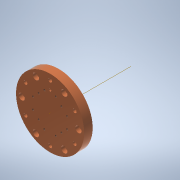
# Autodesk Inventor part: base_becherboden
Saved by Autodesk Inventor 2020 (Build 240168000, 168)
## iProperties
Created: 2018-08-22
Part Number: base_becherboden
Material: ABS Plastic
Document SubType Name: Modeling
Designer: Q
Density: 1.06 g/cm^3
Appearance: Smooth - White
Mass: 1439.4 g
Surface Area: 317.494 cm^2
Volume: 161.006 cm^3
Author: Q
Autodesk Inventor part; units mm, degrees
ref_plane "YZ Plane" through (0, 0, 0) normal (1, 0, 0) x (0, 1, 0)
ref_plane "XZ Plane" through (0, 0, 0) normal (0, 1, 0) x (-1, 0, 0)
ref_plane "XY Plane" through (0, 0, 0) normal (0, 0, 1) x (1, 0, 0)
sketch "Sketch1" plane through (0, 0, 0) normal (0, 0, 1) x (1, 0, 0)
  circle A0 centre (0, 0) radius 60 projected
  point P0 (0, 0)
  point P1 (-51.3571, -31.5041)
  point P2 (-31.5041, -51.3571)
  constraints: 1 other
extrude "Extrusion1" add sketch "Sketch1" along normal blind 15
sketch "Sketch13" plane through (0, 0, 0) normal (0, 0, -1) x (-1, 0, 0)
  point P0 (0, 0)
  point P1 (0, 0)
  constraints: 1 coincident
sketch "Sketch14" plane through (0, 0, 15) normal (0, 0, 1) x (1, 0, 0)
  circle A0 centre (0, 50) radius 2.4585 projected
  point P0 (0, 0)
hole "Hole10" at (0, 50, 15) direction (0, 0, -1) diameter 6.6 depth 17.1 clearance for "Socket Head Cap Screw ISO 4762" size "M6" standard "ISO"
pattern_circular "Circular Pattern6" count 6 over 360 about axis through (0, 0, 0) along (0, 0, 1) of "Hole10"
sketch "Sketch15" plane through (0, 0, 15) normal (0, 0, 1) x (1, 0, 0)
  circle A0 centre (25, 43.3013) radius 2.4585 projected
  point P0 (0, 0)
hole "Hole11" at (25, 43.3013, 15) direction (0, 0, -1) diameter 6.6 end through all counterbore diameter 11 counterbore depth 6.8 clearance for "Socket Head Cap Screw ISO 4762" size "M6" standard "ISO"
pattern_circular "Circular Pattern7" count 6 over 360 about axis through (0, 0, 0) along (0, 0, 1) of "Hole11"
sketch "Sketch16" plane through (0, 0, 0) normal (0, 0, -1) x (-1, 0, 0)
  line L0 (12.05, -6.95) -> (12.05, -3.5) projected
  line L1 (12.05, -3.5) -> (13, -3.5) projected
  line L2 (13, -3.5) -> (13, 6) projected
  line L3 (7, 12) -> (13, 6) projected
  line L4 (7, 12) -> (-7, 12) projected
  line L5 (-13, 6) -> (-7, 12) projected
  line L6 (-13, 6) -> (-13, -3.5) projected
  line L7 (-13, -3.5) -> (-12.05, -3.5) projected
  line L8 (-12.05, -3.5) -> (-12.05, -6.95) projected
  line L9 (-7, -12) -> (-12.05, -6.95) projected
  line L10 (-7, -12) -> (7, -12) projected
  line L11 (12.05, -6.95) -> (7, -12) projected
  circle A0 centre (-10, -5.5) radius 1.35 projected
  circle A1 centre (10, -5.5) radius 1.35 projected
  circle A2 centre (-10, 5.5) radius 0.8 projected
  circle A3 centre (10, 5.5) radius 0.8 projected
  point P0 (0, 0)
hole "Hole12" at (10, -5.5, 0) at (-10, -5.5, 0) direction (0, 0, 1) diameter 2.013 depth 7.6 tip angle 118 thread size "M2.5x0.45" class "6H" standard "ISO Metric profile"
sketch "Sketch17" plane through (0, 0, 0) normal (0, 0, -1) x (-1, 0, 0)
  circle A0 centre (-10, 5.5) radius 0.8 projected
  circle A1 centre (10, 5.5) radius 0.8 projected
  point P0 (0, 0)
hole "Hole13" [suppressed]
sketch "Sketch18" plane through (0, 0, 0) normal (0, 0, -1) x (-1, 0, 0)
  circle A0 centre (0, 0) radius 40 projected
  circle A1 centre (0, 0) radius 30 projected
  line L0 (0, 30) -> (0, 40) construction
  circle A2 centre (0, 35) radius 2.5
  point P0 (0, 0)
  dimension "d114" = 5
  constraints: 2 end point, 2 vertical alignment, 1 centre point, 1 midpoint, 1 vertical, 2 other
  measures "d114" diameter of A2
hole "Hole14" at (0, 35, 0) direction (0, 0, 1) diameter 4.134 end through all thread size "M5x0.8" class "6H" standard "ISO Metric profile"
sketch "Sketch20" plane through (0, 0, 0) normal (0, 0, -1) x (-1, 0, 0)
  line L0 (-20, 20) -> (20, 20)
  line L1 (20, 20) -> (20, -20)
  line L2 (20, -20) -> (-20, -20)
  line L3 (-20, -20) -> (-20, 20)
  line L4 (-10, 30) -> (10, 30)
  line L5 (10, 30) -> (10, -30)
  line L6 (10, -30) -> (-10, -30)
  line L7 (-10, -30) -> (-10, 30)
  line L8 (-30, 10) -> (30, 10)
  line L9 (30, 10) -> (30, -10)
  line L10 (30, -10) -> (-30, -10)
  line L11 (-30, -10) -> (-30, 10)
  point P0 (0, 0)
  point P1 (0, 20)
  point P2 (-20, 0)
  point P3 (-20, 0)
  point P4 (0, 20)
  point P5 (20, 0)
  point P6 (0, -20)
  point P7 (-10, 0)
  point P8 (0, 30)
  point P9 (-30, 0)
  point P10 (0, 10)
  dimension "d124" = 40
  dimension "d125" = 40
  dimension "d141" = 60
  dimension "d142" = 20
  dimension "d143" = 20
  dimension "d144" = 60
  constraints: 24 end point, 14 coincident, 8 midpoint, 6 equal length, 3 horizontal, 3 horizontal alignment, 3 vertical alignment, 2 perpendicular, 1 parallel
  measures "d124" distance of L0.start L0.end
  measures "d125" distance of L0.end L1.end
  measures "d141" distance of L6.end L4.start
  measures "d142" distance of L4.start L4.end
  measures "d143" distance of L10.end L8.start
  measures "d144" distance of L8.start L8.end
hole "Hole15" at (20, 20, 0) at (-20, 20, 0) at (-20, -20, 0) at (20, -20, 0) at (30, -10, 0) at (30, 10, 0) at (10, 30, 0) at (-10, 30, 0) at (-30, 10, 0) at (-30, -10, 0) at (-10, -30, 0) at (10, -30, 0) direction (0, 0, 1) diameter 3.3 depth 20 tip angle 118
thread "Thread1" size "M4x0.7" class "6H" standard "ANSI Metric M Profile" full length
thread "Thread2" size "M4x0.7" class "6H" standard "ANSI Metric M Profile" full length
thread "Thread3" size "M4x0.7" class "6H" standard "ANSI Metric M Profile" full length
thread "Thread4" size "M4x0.7" class "6H" standard "ANSI Metric M Profile" full length
thread "Thread5" size "M4x0.7" class "6H" standard "ANSI Metric M Profile" full length
thread "Thread6" size "M4x0.7" class "6H" standard "ANSI Metric M Profile" full length
thread "Thread7" size "M4x0.7" class "6H" standard "ANSI Metric M Profile" full length
thread "Thread8" size "M4x0.7" class "6H" standard "ANSI Metric M Profile" full length
thread "Thread9" size "M4x0.7" class "6H" standard "ANSI Metric M Profile" full length
thread "Thread10" size "M4x0.7" class "6H" standard "ANSI Metric M Profile" full length
thread "Thread11" size "M4x0.7" class "6H" standard "ANSI Metric M Profile" full length
thread "Thread12" size "M4x0.7" class "6H" standard "ANSI Metric M Profile" full length
body "Solid1"
